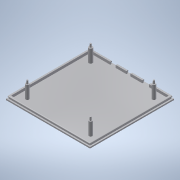
# Autodesk Inventor part: Enclosure_bottom
Saved by Autodesk Inventor 2022.3 (Build 263350000, 350)
## iProperties
Created: 2022-06-20
Part Number: Enclosure_bottom
Material: ABS Plastic
Document SubType Name: Modeling
Designer: abmos
Density: 1.06 g/cm^3
Appearance: Smooth - White
Author: abmos
Autodesk Inventor part; units mm, degrees
ref_plane "YZ Plane" through (0, 0, 0) normal (1, 0, 0) x (0, 1, 0)
ref_plane "XZ Plane" through (0, 0, 0) normal (0, 1, 0) x (-1, 0, 0)
ref_plane "XY Plane" through (0, 0, 0) normal (0, 0, 1) x (1, 0, 0)
sketch "Bottom_profile" plane through (0, 0, 0) normal (0, 1, 0) x (-1, 0, 0)
  line L0 (65, 65) -> (-65, 65)
  line L1 (-65, 65) -> (-65, -65)
  line L2 (-65, -65) -> (65, -65)
  line L3 (65, -65) -> (65, 65)
  line L4 (65, 65) -> (-65, -65) construction
  line L5 (-65, 65) -> (65, -65) construction
  point P0 (0, 0)
  dimension "Enclosure_width" = 130
  dimension "Enclosure_height" = 130
  constraints: 12 end point, 2 midpoint, 2 parallel, 1 horizontal, 1 perpendicular
  measures "Enclosure_width" distance of L2.end L1.end
  measures "Enclosure_height" distance of L1.end L0.end
extrude "Bottom" add sketch "Bottom_profile" along normal blind 2
sketch "Wall_profile" plane through (0, 2, 0) normal (0, 1, 0) x (1, 0, 0)
  line L0 (65, -65) -> (65, 65) projected
  line L1 (65, 65) -> (-65, 65) projected
  line L2 (-65, 65) -> (-65, -65) projected
  line L3 (-65, -65) -> (65, -65) projected
  line L4 (-63, 63) -> (63, 63)
  line L5 (63, 63) -> (63, -63)
  line L6 (63, -63) -> (-63, -63)
  line L7 (-63, -63) -> (-63, 63)
  line L8 (61, 61) -> (-61, 61)
  line L9 (-61, 61) -> (-61, -61)
  line L10 (-61, -61) -> (61, -61)
  line L11 (61, -61) -> (61, 61)
  point P0 (0, 0)
  dimension "Wall_from_outer" = 2
  dimension "Wall_thickness" = 2
  constraints: 16 end point, 6 other
  measures "Wall_from_outer" distance between parallel lines of L1 L4
  measures "Wall_thickness" distance between parallel lines of L4 L8
extrude "Walls" add sketch "Wall_profile" along normal blind 4 contours L4 L5 L6 L7
sketch "Lip_front_profile" plane through (63, 2, 63) normal (1, 0, 0) x (0, 0, -1)
  line L0 (0, 0) -> (0, 4) projected
  arc A0 (0, 4) -> (0, 2) centre (0, 3) ccw
  line L1 (0, 3) -> (0, 4) construction
  line L2 (0, 3) -> (1, 3) construction
  line L3 (0, 3) -> (0, 2) construction
  line L4 (0, 4) -> (126, 4) projected
  line L5 (2, 4) -> (124, 4) construction
  line L6 (128, 0) -> (-2, 0) construction
  point P0 (63, -2)
  point P1 (0, 4)
  point P2 (0, 2)
  dimension "Lip_diameter" = 1
  dimension "d9" = 90
  dimension "d10" = 180
  dimension "d11" = 1
  constraints: 6 end point, 2 point on circle, 1 centre point, 1 horizontal, 1 perpendicular, 1 point on line
  measures "Lip_diameter" radius of A0
  measures "d9" angle of L2 L1
  measures "d10" angle of L3 L1
  measures "d11" distance from line of L4 L1.start
extrude "Lip_front" add sketch "Lip_front_profile" against normal up to surface (126 mm away)
revolve "Lip_corner" add sketch "Lip_front_profile" angle 90 about axis through (63, 2, 63) along (0, 1, 0)
pattern_circular "Lip_mirroring" count 4 over 360 about axis through (0, -10, 0) along (0, 1, 0) of "Lip_front", "Lip_corner"
sketch "PCB_mounting_holes" plane through (0, 2, 0) normal (0, 1, 0) x (1, 0, 0)
  ellipse E0 centre (49.4971, -48.607) end of major axis (48.1662, -47.7189) minor radius 1.6 projected
  ellipse E1 centre (-48.5028, -48.5929) end of major axis (-49.8337, -47.7048) minor radius 1.6 projected
  ellipse E2 centre (49.5112, 49.393) end of major axis (48.1803, 50.2811) minor radius 1.6 projected
  ellipse E3 centre (-48.4888, 49.4071) end of major axis (-49.8197, 50.2952) minor radius 1.6 projected
  point P0 (0, 0)
  constraints: 4 other
extrude "PCB_post_inner" add sketch "PCB_mounting_holes" along normal blind 25 draft -1
sketch "PCB_post_outer_offsets" plane through (0, 2, 0) normal (0, 1, 0) x (1, 0, 0)
  circle A0 centre (-48.4879, 49.4084) radius 1.6 projected
  circle A1 centre (-48.4879, -48.5916) radius 1.6 projected
  circle A2 centre (49.5121, -48.5916) radius 1.6 projected
  circle A3 centre (49.5121, 49.4084) radius 1.6 projected
  circle A4 centre (-48.4879, 49.4084) radius 2.6
  circle A5 centre (-48.4879, 49.4084) radius 2.952
  circle A6 centre (-48.4879, -48.5916) radius 2.6
  circle A7 centre (49.5121, -48.5916) radius 2.6
  circle A8 centre (49.5121, 49.4084) radius 2.6
  point P0 (0, 0)
  dimension "d26" = 1
  dimension "d27" = 1
  dimension "d29" = 1
  dimension "d30" = 1
  constraints: 5 centre point
  measures "d26" radial gap between concentric circles of A0 A4
  measures "d27" radial gap between concentric circles of A1 A6
  measures "d29" radial gap between concentric circles of A3 A8
  measures "d30" radial gap between concentric circles of A2 A7
extrude "PCB_post_outer" add sketch "PCB_post_outer_offsets" along normal blind 20 contours A0 | A1 | A2 | A3 | A4 | A5 | A6 | A7 | A8
sketch "Sketch8" plane through (0, 6, 0) normal (0, 1, 0) x (1, 0, 0)
  line L0 (30.32, 60.0205) -> (19.9076, 60.0205)
  line L1 (19.9076, 60.0205) -> (19.9076, 65.3385)
  line L2 (19.9076, 65.3385) -> (30.32, 65.3385)
  line L3 (30.32, 65.3385) -> (30.32, 60.0205)
  line L4 (1.6581, 60.0205) -> (-4.6585, 60.0205)
  line L5 (-4.6585, 60.0205) -> (-4.6585, 65.3385)
  line L6 (-4.6585, 65.3385) -> (1.6581, 65.3385)
  line L7 (1.6581, 65.3385) -> (1.6581, 60.0205)
  line L8 (-21.1609, 60.0205) -> (-29.7673, 60.0205)
  line L9 (-29.7673, 60.0205) -> (-29.7673, 65.3385)
  line L10 (-29.7673, 65.3385) -> (-21.1609, 65.3385)
  line L11 (-21.1609, 65.3385) -> (-21.1609, 60.0205)
  point P0 (0, 0)
  constraints: 24 end point, 6 parallel, 4 point on line, 3 horizontal, 3 perpendicular
extrude "Extrusion7" cut sketch "Sketch8" against normal blind 4
equation "\"d11\" = Lip_diameter"
equation "\"d27\" = d26"
equation "\"d29\" = d26"
equation "\"d30\" = d26"
body "Solid1"
